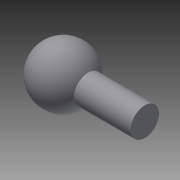
# Autodesk Inventor part: ball joint ball
Saved by Autodesk Inventor 2015 SP2 (Build 190223200, 223)
## iProperties
Created: 2015-05-24
Part Number: ball joint ball
Material: Generic
Document SubType Name: Modeling
Designer: caleb
Density: 1 g/cm^3
Appearance: Default
Author: caleb
Autodesk Inventor part; units mm, degrees
ref_plane "YZ Plane" through (0, 0, 0) normal (1, 0, 0) x (0, 1, 0)
ref_plane "XZ Plane" through (0, 0, 0) normal (0, 1, 0) x (-1, 0, 0)
ref_plane "XY Plane" through (0, 0, 0) normal (0, 0, 1) x (1, 0, 0)
sketch "Sketch1" plane through (0, 0, 0) normal (0, 1, 0) x (-1, 0, 0)
  line L0 (0, 0) -> (24.5493, 0)
  arc A0 (12.7, -3.175) -> (24.5493, 0) centre (18.1993, 0) ccw
  line L1 (12.7, -3.175) -> (0, -3.175)
  line L2 (0, -3.175) -> (0, 0)
  dimension "d0" = 3.175
  dimension "d1" = 6.35
  dimension "d2" = 12.7
  constraints: 6 end point, 2 point on circle, 1 centre point, 1 horizontal, 1 parallel, 1 perpendicular, 1 point on line
  measures "d0" distance of L1.end L0.start
  measures "d1" radius of A0
  measures "d2" distance of L1.start L1.end
revolve "Revolution1" add sketch "Sketch1" angle 360 about axis through (0, 0, 0) along (-1, 0, 0)
body "Solid1"
